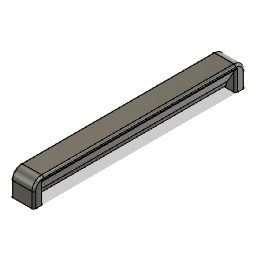
CoatingBlade-0p75mm (Autodesk Fusion 360 design; units mm, degrees)
Autodesk Fusion 360 part; units mm, degrees
note: some values were not read from the file. Chosen so that the rebuilt part matches the saved one: which face or edge a step refers to; which pieces of a blend or face edit are solid.
sketch "Sketch1" plane through (0, 0, 0) normal (0, 1, 0) x (1, 0, 0)
  line L0 (1, -50) -> (-1, -50)
  line L1 (-1, -50) -> (-1, 50)
  line L2 (-1, 50) -> (1, 50)
  line L3 (1, 50) -> (1, -50)
  line L4 (1, -50) -> (-1, 50) construction
  line L5 (-1, -50) -> (1, 50) construction
  line L6 (-6, -50) -> (6, -50)
  line L7 (6, -50) -> (6, -55)
  line L8 (6, -55) -> (-6, -55)
  line L9 (-6, -55) -> (-6, -50)
  line L10 (-6, 0) -> (6, 0)
  line L11 (6, 55) -> (-6, 55)
  line L12 (-6, 55) -> (-6, 50)
  line L13 (-6, 50) -> (6, 50)
  line L14 (6, 50) -> (6, 55)
  dimension "d1" = 100
  dimension "d2" = 2
  dimension "d3" = 12
  dimension "d4" = 5
  dimension "d5" = 5
  dimension "d6" = 5
  constraint perpendicular L0 L1
  constraint parallel L0 L2
  constraint parallel L1 L3
  constraint horizontal L0
  constraint coincident L4 origin
  constraint coincident L5 origin
  constraint horizontal L6
  constraint vertical L7
  constraint horizontal L8
  constraint vertical L9
  constraint perpendicular L1 L10
  constraint symmetric L6.start L10 L12.end
  constraint symmetric L6.end L10 L13.end
  constraint symmetric L7.end L10 L11.start
  constraint symmetric L8.end L10 L11.end
  measures "d1" distance of L0.end L1.end
  measures "d2" distance of L1.end L2.end
  measures "d3" distance of L6.start L6.end
  measures "d4" distance of L6.start L8.end
  measures "d5" distance of L1 L6.start
  measures "d6" distance of L0.start L6.end
extrude "Extrude1" add sketch "Sketch1" along normal blind 10
sketch "Sketch2" plane through (0, 0, 0) normal (0, -1, 0) x (1, 0, 0)
  line L0 (6, -50) -> (1, -50)
  line L1 (1, -50) -> (1, 50)
  line L2 (1, 50) -> (6, 50)
  line L3 (6, 50) -> (6, 55)
  line L4 (6, 55) -> (-6, 55)
  line L5 (-6, 55) -> (-6, 50)
  line L6 (-6, 50) -> (-1, 50)
  line L7 (-1, 50) -> (-1, -50)
  line L8 (-1, -50) -> (-6, -50)
  line L9 (-6, -50) -> (-6, -55)
  line L10 (-6, -55) -> (6, -55)
  line L11 (6, -55) -> (6, -50)
  line L12 (-6, 55) -> (6, 55)
  line L13 (6, 55) -> (6, 50)
  line L14 (6, 50) -> (-6, 50)
  line L15 (-6, 50) -> (-6, 55)
  line L16 (-6, -50) -> (6, -50)
  line L17 (6, -50) -> (6, -55)
  line L18 (6, -55) -> (-6, -55)
  line L19 (-6, -55) -> (-6, -50)
  constraint horizontal L12
  constraint vertical L13
  constraint horizontal L14
  constraint vertical L15
  constraint coincident L2.end L3.start
  constraint coincident L4.end L5.start
  constraint horizontal L16
  constraint vertical L17
  constraint horizontal L18
  constraint vertical L19
  constraint coincident L10.end L11.start
  constraint coincident L8.end L9.start
extrude "Extrude2" add sketch "Sketch2" along normal blind 0.75 contours L0 L8 L9 L10 L11 L16 L17 L18 L19 | L2 L3 L4 L5 L6 L12 L13 L14 L15
sketch "Sketch3" plane through (0, 10, 0) normal (0, 1, 0) x (-1, 0, 0)
  line L0 (-1, -50) -> (-6, -50)
  line L1 (-6, -50) -> (-6, -55)
  line L2 (-6, -55) -> (6, -55)
  line L3 (6, -55) -> (6, -50)
  line L4 (6, -50) -> (1, -50)
  line L5 (1, -50) -> (1, 50)
  line L6 (1, 50) -> (6, 50)
  line L7 (6, 50) -> (6, 55)
  line L8 (6, 55) -> (-6, 55)
  line L9 (-6, 55) -> (-6, 50)
  line L10 (-6, 50) -> (-1, 50)
  line L11 (-1, 50) -> (-1, -50)
  line L12 (6, 55) -> (-6, 55)
  line L13 (-6, 55) -> (-6, -55)
  line L14 (-6, -55) -> (6, -55)
  line L15 (6, -55) -> (6, 55)
  constraint horizontal L12
  constraint vertical L13
  constraint horizontal L14
  constraint vertical L15
  constraint coincident L1.end L2.start
  constraint coincident L7.end L8.start
extrude "Extrude3" add sketch "Sketch3" along normal blind 2
chamfer "Chamfer1" distance 5 angle 60 2 edges at (-1, 10, 0) (1, 10, 0) measured on face at (-2.6667, 10, 16.6667) measured on face at (2.6667, 10, -16.6667)
fillet "Fillet1" radius 5 2 edges at (1, 1.3397, 0) (-1, 1.3397, 0)
fillet "Fillet2" radius 5 2 edges at (0, 12, 55) (0, 12, -55)
fillet "Fillet3" radius 1 14 edges at (6, 3.125, 55) (6, 10.5355, 53.5355) (6, 12, 0) (6, 10.5355, -53.5355) (6, 10, 0) (6, 3.125, -55) (-6, 3.125, 55) (-6, 10.5355, 53.5355) (-6, 12, 0) (-6, 10.5355, -53.5355) (5.999, 10, 0) (-6, 3.125, -55) (-6, 10, 0) (-5.999, 10, 0)
fillet "Fillet4" radius 1 4 edges at (6, 4.759, -50) (-6, 4.759, -50) (-6, 4.759, 50) (6, 4.759, 50)
fillet "Fillet5" radius 0.5 2 edges at (0, 0, 50) (0, 0, -50)
fillet "Fillet6" radius 0.25 6 edges at (-1.0022, -0.1467, 49.8538) (-1, 0, 0) (-1.0022, -0.1467, -49.8538) (1.0022, -0.1467, -49.8538) (1, 0, 0) (1.0022, -0.1467, 49.8538)
